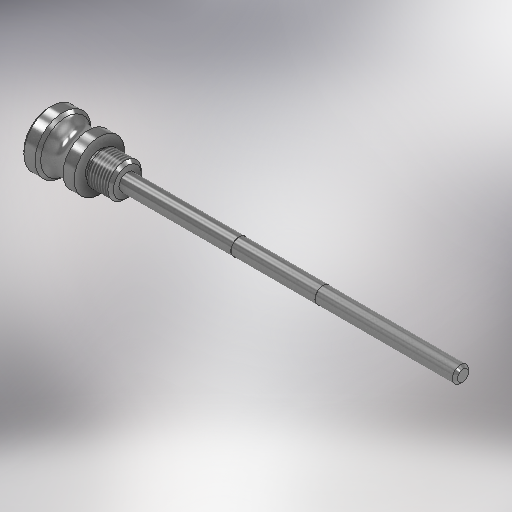
# Autodesk Inventor part: 杆式油标
Saved by Autodesk Inventor 2025 (Build 290162000, 162)
## iProperties
Created: 2025-03-14
Part Number: 杆式油标
Material: 钢，软
Document SubType Name: Modeling
Designer: ASUS
Density: 7.85 g/cm^3
Appearance: 磨光 - 深灰色
Author: ASUS
Autodesk Inventor part; units mm, degrees
ref_plane "YZ Plane" through (0, 0, 0) normal (1, 0, 0) x (0, 1, 0)
sketch "草图1" plane through (0, 0, 0) normal (0, 1, 0) x (-1, 0, 0)
  line L0 (0, 0) -> (0, 9)
  line L1 (0, 9) -> (-1, 10)
  line L2 (-1, 10) -> (-5, 10)
  line L3 (-5, 10) -> (-6, 9)
  line L4 (29.6, 0) -> (-177.6, 0) projected
  arc A0 (-14, 9) -> (-6, 9) centre (-10, 13) ccw
  line L5 (-14, 9) -> (-18, 9)
  line L6 (-18, 9) -> (-18, 5)
  line L7 (-18, 5) -> (-19.5, 5)
  line L8 (-19.5, 5) -> (-19.5, 6)
  line L9 (-19.5, 6) -> (-27, 6)
  line L10 (-27, 6) -> (-28, 5)
  line L11 (-28, 5) -> (-28, 3)
  line L12 (-28, 3) -> (-147, 3)
  line L13 (0, 0) -> (-118, 0)
  line L14 (-147, 3) -> (-148, 2)
  line L15 (-148, 2) -> (-148, 0)
  dimension "d0" = 10
  dimension "d4" = 45
  dimension "d5" = 1
  dimension "d6" = 45
  dimension "d7" = 1
  dimension "d8" = 6
  dimension "d9" = 6
  dimension "d10" = 45
  dimension "d11" = 1
  dimension "d12" = 3
  dimension "d13" = 4
  dimension "d14" = 10
  dimension "d16" = 28
  dimension "d17" = 9
  dimension "d18" = 1.5
  dimension "d19" = 1
  dimension "d21" = 45
  dimension "d22" = 1
  dimension "d23" = 130
  constraints: 30 end point, 7 perpendicular, 2 point on circle, 2 point on line, 1 centre point, 1 horizontal, 1 parallel, 1 tangent, 1 vertical
  measures "d0" distance between parallel lines of L4 L2
  measures "d4" angle of L0 L1
  measures "d5" distance from line of L0.end L2
  measures "d6" angle of L2 L3
  measures "d7" distance from line of L3.end L2
  measures "d8" distance from line of L3.end L0
  measures "d9" distance between parallel lines of L13 L9
  measures "d10" angle of L9 L10
  measures "d11" distance from line of L9 L10.end
  measures "d12" distance between parallel lines of L13 L12
  measures "d13" distance of L5.start L5.end
  measures "d14" distance between parallel lines of L11 L6
  measures "d16" distance between parallel lines of L11 L0
  measures "d17" distance between parallel lines of L13 L5
  measures "d18" distance of L6.end L7.end
  measures "d19" distance of L7.end L8.end
  measures "d21" angle of L15 L14
  measures "d22" distance from line of L14.end L12
  measures "d23" distance between parallel lines of L6 L15
revolve "旋转1" add sketch "草图1" angle 360 about axis through (-10, 0, 0) along (1, 0, 0)
thread "螺纹1" size "M12x1" class "4g6g" standard "GB Metric profile" full length
ref_plane "工作平面1" through (98, 0, 0) normal (1, 0, 0) x (0, 0, -1)
sketch "草图2" plane through (98, 0, 0) normal (1, 0, 0) x (0, 0, -1)
  circle A0 centre (0, 0) radius 2.9
  circle A1 centre (0, 0) radius 3
  dimension "d27" = 5.8
  dimension "d30" = 6
  constraints: 2 centre point, 2 coincident
  measures "d27" diameter of A0
  measures "d30" diameter of A1
extrude "拉伸1" cut sketch "草图2" along normal through all
ref_plane "工作平面2" through (68, 0, 0) normal (1, 0, 0) x (0, 0, -1)
sketch "草图3" plane through (68, 0, 0) normal (1, 0, 0) x (0, 0, -1)
  circle A0 centre (0, 0) radius 2.95
  circle A1 centre (0, 0) radius 3
  dimension "d32" = 5.9
  dimension "d33" = 6
  constraints: 2 centre point, 2 coincident
  measures "d32" diameter of A0
  measures "d33" diameter of A1
extrude "拉伸2" cut sketch "草图3" along normal through all
equation "\"d0\" = 0.5 * D"
equation "\"d8\" = b"
equation "\"d9\" = 0.5 * Md"
equation "\"d12\" = 0.5 * d3"
equation "\"d13\" = c_"
equation "\"d14\" = a"
equation "\"d16\" = h_"
equation "\"d23\" = L"
equation "\"d1\" = 4"
equation "\"d2\" = 12"
equation "\"d3\" = 6"
equation "\"h_\" = 28"
equation "\"a\" = 10"
equation "\"b\" = 6"
equation "\"c_\" = 4"
equation "\"D1\" = 16"
equation "\"Md\" = 12"
equation "\"L\" = 130"
equation "\"D\" = 20"
